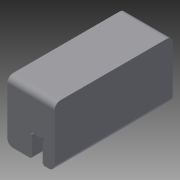
# Autodesk Inventor part: capSenseHolder
Saved by Autodesk Inventor 2015 (Build 190159000, 159)
## iProperties
Created: 2014-12-11
Part Number: capSenseHolder
Material: Generic
Document SubType Name: Modeling
Designer: rawrdong
Density: 1 g/cm^3
Appearance: Default
Author: rawrdong
Autodesk Inventor part; units mm, degrees
ref_plane "YZ Plane" through (0, 0, 0) normal (1, 0, 0) x (0, 1, 0)
ref_plane "XZ Plane" through (0, 0, 0) normal (0, 1, 0) x (-1, 0, 0)
ref_plane "XY Plane" through (0, 0, 0) normal (0, 0, 1) x (1, 0, 0)
sketch "Sketch1" plane through (0, 0, 0) normal (0, 1, 0) x (-1, 0, 0)
  line L0 (0, 0) -> (8, 0)
  line L1 (8, 0) -> (8, -10)
  line L2 (0, -10) -> (0, 0)
  line L3 (3.8, -10) -> (3.8, -6.2)
  line L4 (3.8, -6.2) -> (2, -6.2)
  line L5 (2, -6.2) -> (2, -10)
  line L6 (8, -10) -> (3.8, -10)
  line L7 (2, -10) -> (0, -10)
  dimension "d0" = 1.8
  dimension "d1" = 2
  dimension "d2" = 8
  dimension "d3" = 3.8
  dimension "d4" = 3.8
  dimension "d5" = 10
  constraints: 16 end point, 4 parallel, 2 horizontal, 1 perpendicular, 1 vertical
  measures "d0" distance between parallel lines of L3 L5
  measures "d1" distance of L5.end L2.start
  measures "d2" distance of L0.start L0.end
  measures "d3" distance of L3.start L3.end
  measures "d4" distance of L4.end L5.end
  measures "d5" distance of L2.start L0.start
extrude "Extrusion1" add sketch "Sketch1" along normal blind 20
chamfer "Chamfer1" distance 0.25 angle 45 2 edges at (-2, 10, -10) (-3.8, 10, -10)
fillet "Fillet1" radius 1 4 edges at (-4, 20, 0) (-4, 0, 0) (-8, 10, -10) (0, 10, -10)
sketch "Sketch2" plane through (0, 20, 0) normal (0, 1, 0) x (1, 0, 0)
  arc A0 (0, 9) -> (-1, 10) centre (-1, 9) ccw projected
  line L0 (-1, 10) -> (-1.75, 10) projected
  line L1 (-2, 9.75) -> (-1.75, 10) projected
  line L2 (-2, 9.75) -> (-2, 6.2) projected
  line L3 (-2, 6.2) -> (-3.8, 6.2) projected
  line L4 (-3.8, 6.2) -> (-3.8, 9.75) projected
  line L5 (-4.05, 10) -> (-3.8, 9.75) projected
  line L6 (-4.05, 10) -> (-7, 10) projected
  arc A1 (-7, 10) -> (-8, 9) centre (-7, 9) ccw projected
  line L7 (-8, 9) -> (-8, 1) projected
  line L8 (0, 1) -> (-8, 1) projected
  line L9 (0, 1) -> (0, 9) projected
  circle A2 centre (-3.8, 6.2) radius 0.25
  circle A3 centre (-2, 6.2) radius 0.25
  point P0 (0, 0)
  dimension "d12" = 0.5
  constraints: 2 centre point, 2 coincident, 1 equal radius
  measures "d12" diameter of A2
extrude "Extrusion2" cut sketch "Sketch2" against normal through all contours A3 L3 L2 | L2 L3 A3 | A2 L4 L3 | L3 L4 A2
fillet "Fillet2" radius 0.5 4 edges at (-3.55, 10, -6.2) (-3.8, 10, -6.45) (-2, 10, -6.45) (-2.25, 10, -6.2)
body "Solid1"
